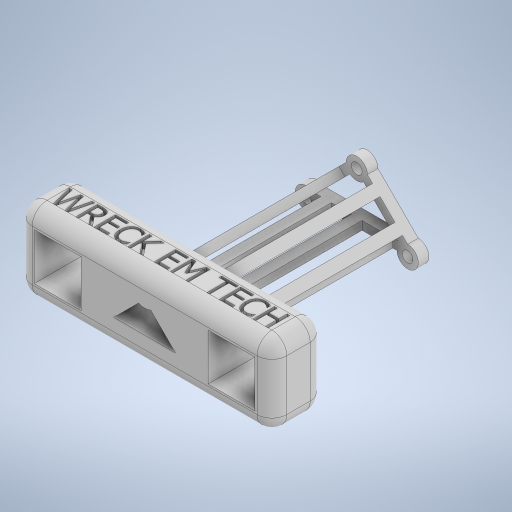
# Autodesk Inventor part: WPNA_FrontHammer
Saved by Autodesk Inventor 2024 (Build 280153000, 153)
## iProperties
Created: 2025-11-09
Part Number: WPNA_FrontHammer
Material: Generic
Document SubType Name: Modeling
Designer: albah
Density: 1 g/cm^3
Appearance: Default
Author: albah
Autodesk Inventor part; units mm, degrees
ref_plane "YZ Plane" through (0, 0, 0) normal (1, 0, 0) x (0, 1, 0)
ref_plane "XZ Plane" through (0, 0, 0) normal (0, 1, 0) x (-1, 0, 0)
sketch "Sketch1" plane through (0, 0, 0) normal (0, 0, 1) x (1, 0, 0)
  line L0 (0, 0) -> (24, 0)
  line L1 (0, 0) -> (-24, 0)
  line L2 (0, 0) -> (0, 24)
  circle A0 centre (0, 24) radius 2.5
  circle A1 centre (24, 0) radius 2.5
  circle A2 centre (-24, 0) radius 2.5
  circle A3 centre (0, 24) radius 5
  circle A4 centre (-24, 0) radius 5
  circle A5 centre (24, 0) radius 5
  line L3 (-24, 5) -> (-5, 24)
  line L4 (5, 24) -> (24, 5)
  line L5 (2.1716, 21.1716) -> (21.1716, 2.1716)
  line L6 (-21.1716, 2.1716) -> (-2.1716, 21.1716)
  line L7 (0, 4) -> (24, 4)
  line L8 (0, 4) -> (-24, 4)
  line L9 (-20.5858, 8.4142) -> (-17.7574, 5.5858)
  line L10 (-17.7574, 5.5858) -> (-14.2218, 9.1213)
  line L11 (-14.2218, 9.1213) -> (-17.0503, 11.9497)
  line L12 (-17.0503, 11.9497) -> (-20.5858, 8.4142)
  line L13 (-11.9497, 17.0503) -> (-9.1213, 14.2218)
  line L14 (-9.1213, 14.2218) -> (-5.5858, 17.7574)
  line L15 (-5.5858, 17.7574) -> (-8.4142, 20.5858)
  line L16 (-8.4142, 20.5858) -> (-11.9497, 17.0503)
  line L17 (7.4497, 21.5503) -> (4.6213, 18.7218)
  line L18 (4.6213, 18.7218) -> (8.1569, 15.1863)
  line L19 (8.1569, 15.1863) -> (10.9853, 18.0147)
  line L20 (10.9853, 18.0147) -> (7.4497, 21.5503)
  line L21 (21.5503, 7.4497) -> (18.7218, 4.6213)
  line L22 (18.7218, 4.6213) -> (15.1863, 8.1569)
  line L23 (15.1863, 8.1569) -> (18.0147, 10.9853)
  line L24 (18.0147, 10.9853) -> (21.5503, 7.4497)
  line L25 (17, 4) -> (17, 0)
  line L26 (17, 0) -> (12, 0)
  line L27 (12, 0) -> (12, 4)
  line L28 (12, 4) -> (17, 4)
  line L29 (1.1005, 0) -> (-3.8995, 0)
  line L30 (-3.8995, 4) -> (1.1005, 4)
  line L31 (-12, 4) -> (-12, 0)
  line L32 (-12, 0) -> (-17, 0)
  line L33 (-17, 0) -> (-17, 4)
  line L34 (-17, 4) -> (-12, 4)
  line L35 (-2.5, 0) -> (2.5, 0)
  line L36 (2.5, 0) -> (2.5, 4)
  line L37 (2.5, 4) -> (-2.5, 4)
  line L38 (-2.5, 4) -> (-2.5, 0)
  line L39 (-2.5, 0) -> (2.5, 4) construction
  line L40 (2.5, 0) -> (-2.5, 4) construction
  point P0 (-7, 19.1716)
  point P1 (-19.1716, 7)
  point P2 (0, 2)
  point P3 (-3.1918, 20.1513)
  point P4 (-19, 0)
  point P5 (19, 0)
  point P6 (3.1918, 20.1513)
  point P7 (19.3431, 4)
  point P8 (-19.3431, 4)
  dimension "d7" = 10
  dimension "d0" = 24
  dimension "d1" = 24
  dimension "d2" = 24
  dimension "d3" = 5
  dimension "d4" = 5
  dimension "d5" = 5
  dimension "d6" = 10
  dimension "d8" = 10
  dimension "d9" = 4
  dimension "d10" = 4
  dimension "d11" = 4
  dimension "d12" = 4
  dimension "d13" = 45
  dimension "d14" = 20.5061
  dimension "d15" = 16.5061
  dimension "d16" = 1
  dimension "d17" = 0.7071
  dimension "d18" = 1.8284
  dimension "d19" = 17.1716
  dimension "d20" = 17.6777
  dimension "d21" = 17.6777
  dimension "d22" = 7.0711
  dimension "d23" = 33.9411
  dimension "d24" = 34.6482
  dimension "d27" = 5
  dimension "d28" = 5
  dimension "d29" = 5
  dimension "d30" = 5
  dimension "d31" = 5
  dimension "d32" = 5
  dimension "d33" = 5
  dimension "d34" = 7
  dimension "d35" = 7
  dimension "d36" = 7
  dimension "d37" = 7
  dimension "d38" = 5
  dimension "d39" = 7
  dimension "d40" = 7
  dimension "d41" = 6.34
  dimension "d42" = 135
  dimension "d43" = 0
  dimension "d44" = 9.1924
  dimension "d45" = 15.5564
  constraints: 82 end point, 19 parallel, 15 perpendicular, 14 point on line, 6 coincident, 6 midpoint, 5 centre point, 2 horizontal, 2 point on circle, 1 vertical, 3 other
  measures "d0" distance of L0.start L0.end
  measures "d1" distance of L0.start L1.end
  measures "d2" distance of L0.start L2.end
  measures "d3" diameter of A0
  measures "d4" diameter of A1
  measures "d5" diameter of A2
  measures "d6" diameter of A3
  measures "d8" diameter of A5
  measures "d9" distance between parallel lines of L4 L5
  measures "d10" distance between parallel lines of L3 L6
  measures "d11" distance between parallel lines of L0 L7
  measures "d12" distance between parallel lines of L1 L8
  measures "d13" angle of L7 L4
  measures "d14" distance from line of L0.start L4
  measures "d15" distance from line of L0.start L6
  measures "d16" distance from line of L4.end L7
  measures "d17" distance from line of L7.end L4
  measures "d18" distance from line of L5.end L7
  measures "d19" distance from line of L5.start L7
  measures "d20" distance from line of L7.start L4
  measures "d21" distance from line of L8.start L4
  measures "d22" distance from line of L6.end L4
  measures "d23" distance from line of L6.start L4
  measures "d24" distance from line of L8.end L4
  measures "d27" distance of L10.end L9.end
  measures "d28" distance of L14.end L13.end
  measures "d29" distance of L18.end L17.end
  measures "d30" distance of L21.end L22.end
  measures "d31" distance of L25.end L26.end
  measures "d32" distance of L29.start L29.end
  measures "d33" distance of L31.end L32.end
  measures "d34" horizontal distance of A3.centre point (-7, 19.172)
  measures "d35" vertical distance of point (-24, 0) point (-19.172, 7)
  measures "d36" distance from line of point (-24, 0) L33
  measures "d37" distance from line of A5.centre L25
  measures "d38" distance of L35.start L35.end
  measures "d39" distance from line of A5.centre L21
  measures "d40" distance from line of A3.centre L17
  measures "d41" angle of L21 L39
  measures "d42" angle of L30 L21
  measures "d43" distance between parallel lines of L7 L37
  measures "d44" distance from line of L29.start L21
  measures "d45" distance from line of L30.start L21
extrude "Extrusion1" add sketch "Sketch1" along normal blind 5 contours L2 L7 L36 L0 | L1 L38 L8 L2 | L1 L31 L8 L38 | L36 L7 L27 L0 | A3 | L27 L7 L25 L0 | L1 L33 L8 L31 | L6 L15 L3 A3 | A3 L4 L17 L5 | L25 L7 L5 A5 L0 | L1 A4 L6 L8 L33 | L6 L13 L3 L15 | L17 L4 L19 L5 | A5 | A4 | L6 L11 L3 L13 | L19 L4 L23 L5 | L5 L7 A5 | L5 L21 L4 A5 L7 | L3 L9 L6 L8 A4 | A4 L8 L6 | L6 L9 L3 L11 | L23 L4 L21 L5
extrude "Extrusion2" add sketch "Sketch1" along normal blind 80 contours L2 L7 L36 L0 | L1 L38 L8 L2 | L27 L7 L25 L0 | L1 L33 L8 L31 | L6 L13 L3 L15 | L17 L4 L19 L5 | L6 L9 L3 L11 | L23 L4 L21 L5
sketch "Sketch2" plane through (0, 0, 80) normal (0, 0, 1) x (1, 0, 0)
  arc A0 (-24, 5) -> (-19, 0) centre (-24, 0) ccw projected
  line L0 (-24, -5) -> (24, -5)
  arc A1 (19, 0) -> (24, 5) centre (24, 0) ccw projected
  line L1 (0, -5) -> (0, 29)
  arc A2 (5, 24) -> (-5, 24) centre (0, 24) ccw projected
  line L2 (-60, -7) -> (60, -7)
  line L3 (60, -7) -> (60, 31)
  line L4 (60, 31) -> (-60, 31)
  line L5 (-60, 31) -> (-60, -7)
  line L6 (-60, -7) -> (60, 31) construction
  line L7 (60, -7) -> (-60, 31) construction
  point P0 (0, 0)
  point P1 (0, 12)
  dimension "d48" = 120
  dimension "d49" = 38
  constraints: 16 end point, 4 midpoint, 3 perpendicular, 3 point on circle, 2 parallel, 2 tangent
  measures "d48" distance of L2.start L2.end
  measures "d49" distance of L3.end L2.end
extrude "Extrusion3" add sketch "Sketch2" along normal blind 25
sketch "Sketch3" plane through (0, 0, 80) normal (0, 0, -1) x (-1, 0, 0)
  line L0 (30, 23) -> (30, 1)
  line L1 (30, 1) -> (52, 1)
  line L2 (52, 1) -> (52, 23)
  line L3 (52, 23) -> (30, 23)
  line L4 (30, 23) -> (52, 1) construction
  line L5 (30, 1) -> (52, 23) construction
  line L6 (60, 31) -> (60, -7) projected
  line L7 (-60, 31) -> (60, 31) projected
  line L8 (60, -7) -> (-60, -7) projected
  line L9 (-52, 23) -> (-30, 23)
  line L10 (-30, 23) -> (-30, 1)
  line L11 (-30, 1) -> (-52, 1)
  line L12 (-52, 1) -> (-52, 23)
  line L13 (-52, 23) -> (-30, 1) construction
  line L14 (-30, 23) -> (-52, 1) construction
  line L15 (-60, -7) -> (-60, 31) projected
  line L16 (-19.3431, 4) -> (19.3431, 4) projected
  line L17 (-3.1918, 20.1513) -> (-4.6213, 18.7218) projected
  line L18 (-3.1918, 20.1513) -> (-19.3431, 4)
  line L19 (-19.3431, 4) -> (19.3431, 4)
  line L20 (19.3431, 4) -> (3.1918, 20.1513)
  arc A0 (-3.1918, 20.1513) -> (3.1918, 20.1513) centre (0, 24) ccw projected
  arc A1 (-3.1918, 20.1513) -> (3.1918, 20.1513) centre (0, 24) ccw
  line L21 (-14.5147, 6) -> (-2.8902, 17.6245)
  arc A2 (-2.8902, 17.6245) -> (2.8902, 17.6245) centre (0, 24) ccw
  line L22 (2.8902, 17.6245) -> (14.5147, 6)
  line L23 (14.5147, 6) -> (-14.5147, 6)
  point P0 (0, 0)
  point P1 (41, 12)
  point P2 (-41, 12)
  point P3 (0, 4)
  point P4 (0, 4)
  dimension "d52" = 8
  dimension "d53" = 8
  dimension "d54" = 8
  dimension "d55" = 8
  dimension "d56" = 8
  dimension "d57" = 8
  dimension "d58" = 30
  dimension "d59" = 30
  dimension "d62" = 2
  constraints: 36 end point, 6 midpoint, 4 parallel, 4 perpendicular, 4 point on circle, 2 centre point, 2 collinear, 1 horizontal, 1 vertical, 3 other
  measures "d52" distance between parallel lines of L6 L2
  measures "d53" distance between parallel lines of L7 L3
  measures "d54" distance between parallel lines of L8 L1
  measures "d55" distance between parallel lines of L8 L11
  measures "d56" distance between parallel lines of L7 L9
  measures "d57" distance between parallel lines of L15 L12
  measures "d58" distance from line of point (0, 4) L0
  measures "d59" distance from line of point (0, 4) L10
  measures "d62" distance between parallel lines of L18 L21
extrude "Extrusion4" cut sketch "Sketch3" against normal blind 25 contours L3 L2 L1 L0 | L9 L10 L11 L12 | L21 A2 L22 L23
fillet "Fillet1" radius 7 12 edges at (60, 12, 80) (0, -7, 80) (-60, 12, 80) (0, 31, 80) (60, -7, 92.5) (0, -7, 105) (-60, -7, 92.5) (-60, 12, 105) (-60, 31, 92.5) (0, 31, 105) (60, 31, 92.5) (60, 12, 105)
fillet "Fillet2" radius 1 25 edges at (6.0355, 20.136, 80) (6.3891, 16.9541, 80) (9.5711, 16.6005, 80) (9.2175, 19.7825, 80) (20.136, 6.0355, 80) (19.7825, 9.2175, 80) (16.6005, 9.5711, 80) (16.9541, 6.3891, 80) (-12, 2, 80) (-14.5, 4, 80) (-17, 2, 80) (17, 2, 80) (14.5, 4, 80) (12, 2, 80) (2.5, 2, 80) (0, 4, 80) (-2.5, 2, 80) (-19.1716, 7, 80) (-15.9896, 7.3536, 80) (-15.636, 10.5355, 80) (-18.818, 10.182, 80) (-10.5355, 15.636, 80) (-7.3536, 15.9896, 80) (-7, 19.1716, 80) (-10.182, 18.818, 80)
ref_plane "Work Plane1" through (-53, 41, 87) normal (0, 1, 0) x (1, 0, 0)
sketch "Sketch7" plane through (-53, 41, 87) normal (0, 1, 0) x (1, 0, 0)
  line L0 (-3.014, -0.6324) -> (108.4129, -0.6324) construction
  line L1 (108.4129, -0.6324) -> (108.4129, -11.6218) construction
  line L2 (108.4129, -11.6218) -> (-3.014, -11.6218) construction
  line L3 (-3.014, -11.6218) -> (-3.014, -0.6324) construction
  line L4 (12.3267, -0.8106) -> (9.8145, -10.8106)
  line L5 (9.8145, -10.8106) -> (8.3234, -10.8106)
  line L6 (8.3234, -10.8106) -> (6.2894, -2.5124)
  line L7 (6.2894, -2.5124) -> (4.3121, -10.8106)
  line L8 (4.3121, -10.8106) -> (2.8372, -10.8106)
  line L9 (2.8372, -10.8106) -> (0.2845, -0.8106)
  line L10 (0.2845, -0.8106) -> (1.6541, -0.8106)
  line L11 (1.6541, -0.8106) -> (3.6638, -9.1008)
  line L12 (3.6638, -9.1008) -> (5.6573, -0.8106)
  line L13 (5.6573, -0.8106) -> (7.0106, -0.8106)
  line L14 (7.0106, -0.8106) -> (9.0203, -9.198)
  line L15 (9.0203, -9.198) -> (11.022, -0.8106)
  line L16 (11.022, -0.8106) -> (12.3267, -0.8106)
  line L17 (21.257, -10.8106) -> (19.5309, -10.8106)
  line L18 (19.5309, -10.8106) -> (16.3704, -6.8317)
  line L19 (16.3704, -6.8317) -> (14.8469, -6.8317)
  line L20 (14.8469, -6.8317) -> (14.8469, -10.8106)
  line L21 (14.8469, -10.8106) -> (13.5179, -10.8106)
  line L22 (13.5179, -10.8106) -> (13.5179, -0.8106)
  line L23 (13.5179, -0.8106) -> (16.0949, -0.8106)
  spline S0 degree 2 poles (16.0949, -0.8106) (16.9539, -0.8106) (18.1127, -0.997) (18.6395, -1.3374) knots 0 0 0 1 2 2 2
  spline S1 degree 2 poles (18.6395, -1.3374) (19.1662, -1.6777) (19.774, -2.7393) (19.774, -3.5254) knots 0 0 0 1 2 2 2
  spline S2 degree 2 poles (19.774, -3.5254) (19.774, -4.6194) (18.6557, -6.1024) (17.6994, -6.4589) knots 0 0 0 1 2 2 2
  line L24 (17.6994, -6.4589) -> (21.257, -10.8106)
  spline S3 degree 2 poles (18.3883, -3.6307) (18.3883, -3.1931) (18.0803, -2.5205) (17.7562, -2.3017) knots 0 0 0 1 2 2 2
  spline S4 degree 2 poles (17.7562, -2.3017) (17.4725, -2.1153) (16.7189, -1.9614) (16.1678, -1.9614) knots 0 0 0 1 2 2 2
  line L25 (16.1678, -1.9614) -> (14.8469, -1.9614)
  line L26 (14.8469, -1.9614) -> (14.8469, -5.7215)
  line L27 (14.8469, -5.7215) -> (16.0139, -5.7215)
  spline S5 degree 2 poles (16.0139, -5.7215) (16.5892, -5.7215) (17.5049, -5.5189) (17.821, -5.2029) knots 0 0 0 1 2 2 2
  spline S6 degree 2 poles (17.821, -5.2029) (18.1127, -4.9273) (18.3883, -4.1494) (18.3883, -3.6307) knots 0 0 0 1 2 2 2
  line L28 (22.0511, -10.8106) -> (22.0511, -0.8106)
  line L29 (22.0511, -0.8106) -> (28.3072, -0.8106)
  line L30 (28.3072, -0.8106) -> (28.3072, -1.9938)
  line L31 (28.3072, -1.9938) -> (23.3801, -1.9938)
  line L32 (23.3801, -1.9938) -> (23.3801, -4.7328)
  line L33 (23.3801, -4.7328) -> (27.975, -4.7328)
  line L34 (27.975, -4.7328) -> (27.975, -5.916)
  line L35 (27.975, -5.916) -> (23.3801, -5.916)
  line L36 (23.3801, -5.916) -> (23.3801, -9.6275)
  line L37 (23.3801, -9.6275) -> (28.3072, -9.6275)
  line L38 (28.3072, -9.6275) -> (28.3072, -10.8106)
  line L39 (28.3072, -10.8106) -> (22.0511, -10.8106)
  spline S7 degree 2 poles (33.6719, -10.9889) (32.6994, -10.9889) (31.0544, -10.3325) (30.4547, -9.6761) knots 0 0 0 1 2 2 2
  spline S8 degree 2 poles (30.4547, -9.6761) (29.855, -9.0278) (29.1986, -7.0829) (29.1986, -5.8187) knots 0 0 0 1 2 2 2
  spline S9 degree 2 poles (29.1986, -5.8187) (29.1986, -4.5627) (29.8388, -2.6988) (30.4466, -2.01) knots 0 0 0 1 2 2 2
  spline S10 degree 2 poles (30.4466, -2.01) (31.0463, -1.3374) (32.6832, -0.6324) (33.6962, -0.6324) knots 0 0 0 1 2 2 2
  spline S11 degree 2 poles (33.6962, -0.6324) (34.1986, -0.6324) (35.0819, -0.7782) (35.4547, -0.8917) knots 0 0 0 1 2 2 2
  spline S12 degree 2 poles (35.4547, -0.8917) (35.7789, -0.997) (36.4515, -1.2969) (36.7837, -1.4751) knots 0 0 0 1 2 2 2
  line L40 (36.7837, -1.4751) -> (36.7837, -3.0797)
  line L41 (36.7837, -3.0797) -> (36.6784, -3.0797)
  spline S13 degree 2 poles (36.6784, -3.0797) (36.5001, -2.9176) (35.949, -2.4638) (35.5519, -2.245) knots 0 0 0 1 2 2 2
  spline S14 degree 2 poles (35.5519, -2.245) (35.1711, -2.0343) (34.2716, -1.7669) (33.6881, -1.7669) knots 0 0 0 1 2 2 2
  spline S15 degree 2 poles (33.6881, -1.7669) (33.0479, -1.7669) (31.9053, -2.2936) (31.4758, -2.7961) knots 0 0 0 1 2 2 2
  spline S16 degree 2 poles (31.4758, -2.7961) (31.0544, -3.3066) (30.5844, -4.8544) (30.5844, -5.8187) knots 0 0 0 1 2 2 2
  spline S17 degree 2 poles (30.5844, -5.8187) (30.5844, -6.8479) (31.0787, -8.3309) (31.5082, -8.8414) knots 0 0 0 1 2 2 2
  spline S18 degree 2 poles (31.5082, -8.8414) (31.9296, -9.3358) (33.056, -9.8382) (33.6881, -9.8382) knots 0 0 0 1 2 2 2
  spline S19 degree 2 poles (33.6881, -9.8382) (34.2635, -9.8382) (35.244, -9.5546) (35.6249, -9.3439) knots 0 0 0 1 2 2 2
  spline S20 degree 2 poles (35.6249, -9.3439) (35.9895, -9.1332) (36.5325, -8.6956) (36.6865, -8.5416) knots 0 0 0 1 2 2 2
  line L42 (36.6865, -8.5416) -> (36.7837, -8.5416)
  line L43 (36.7837, -8.5416) -> (36.7837, -10.1299)
  spline S21 degree 2 poles (36.7837, -10.1299) (36.4515, -10.2839) (35.868, -10.5675) (35.4547, -10.6972) knots 0 0 0 1 2 2 2
  spline S22 degree 2 poles (35.4547, -10.6972) (35.0171, -10.8431) (34.2716, -10.9889) (33.6719, -10.9889) knots 0 0 0 1 2 2 2
  line L44 (45.3169, -10.8106) -> (43.5908, -10.8106)
  line L45 (43.5908, -10.8106) -> (39.9361, -6.1591)
  line L46 (39.9361, -6.1591) -> (39.3526, -6.8155)
  line L47 (39.3526, -6.8155) -> (39.3526, -10.8106)
  line L48 (39.3526, -10.8106) -> (38.0236, -10.8106)
  line L49 (38.0236, -10.8106) -> (38.0236, -0.8106)
  line L50 (38.0236, -0.8106) -> (39.3526, -0.8106)
  line L51 (39.3526, -0.8106) -> (39.3526, -5.4055)
  line L52 (39.3526, -5.4055) -> (43.4531, -0.8106)
  line L53 (43.4531, -0.8106) -> (45.0738, -0.8106)
  line L54 (45.0738, -0.8106) -> (40.9328, -5.2758)
  line L55 (40.9328, -5.2758) -> (45.3169, -10.8106)
  line L56 (50.4061, -10.8106) -> (50.4061, -0.8106)
  line L57 (50.4061, -0.8106) -> (56.6622, -0.8106)
  line L58 (56.6622, -0.8106) -> (56.6622, -1.9938)
  line L59 (56.6622, -1.9938) -> (51.7351, -1.9938)
  line L60 (51.7351, -1.9938) -> (51.7351, -4.7328)
  line L61 (51.7351, -4.7328) -> (56.3299, -4.7328)
  line L62 (56.3299, -4.7328) -> (56.3299, -5.916)
  line L63 (56.3299, -5.916) -> (51.7351, -5.916)
  line L64 (51.7351, -5.916) -> (51.7351, -9.6275)
  line L65 (51.7351, -9.6275) -> (56.6622, -9.6275)
  line L66 (56.6622, -9.6275) -> (56.6622, -10.8106)
  line L67 (56.6622, -10.8106) -> (50.4061, -10.8106)
  line L68 (66.6946, -10.8106) -> (65.3656, -10.8106)
  line L69 (65.3656, -10.8106) -> (65.3656, -2.1964)
  line L70 (65.3656, -2.1964) -> (62.7562, -8.0554)
  line L71 (62.7562, -8.0554) -> (61.9458, -8.0554)
  line L72 (61.9458, -8.0554) -> (59.3607, -2.1964)
  line L73 (59.3607, -2.1964) -> (59.3607, -10.8106)
  line L74 (59.3607, -10.8106) -> (58.1208, -10.8106)
  line L75 (58.1208, -10.8106) -> (58.1208, -0.8106)
  line L76 (58.1208, -0.8106) -> (59.9361, -0.8106)
  line L77 (59.9361, -0.8106) -> (62.432, -6.3779)
  line L78 (62.432, -6.3779) -> (64.8469, -0.8106)
  line L79 (64.8469, -0.8106) -> (66.6946, -0.8106)
  line L80 (66.6946, -0.8106) -> (66.6946, -10.8106)
  line L81 (75.3494, -10.8106) -> (75.3494, -1.9938)
  line L82 (75.3494, -1.9938) -> (71.9944, -1.9938)
  line L83 (71.9944, -1.9938) -> (71.9944, -0.8106)
  line L84 (71.9944, -0.8106) -> (80.0333, -0.8106)
  line L85 (80.0333, -0.8106) -> (80.0333, -1.9938)
  line L86 (80.0333, -1.9938) -> (76.6784, -1.9938)
  line L87 (76.6784, -1.9938) -> (76.6784, -10.8106)
  line L88 (76.6784, -10.8106) -> (75.3494, -10.8106)
  line L89 (81.0463, -10.8106) -> (81.0463, -0.8106)
  line L90 (81.0463, -0.8106) -> (87.3024, -0.8106)
  line L91 (87.3024, -0.8106) -> (87.3024, -1.9938)
  line L92 (87.3024, -1.9938) -> (82.3753, -1.9938)
  line L93 (82.3753, -1.9938) -> (82.3753, -4.7328)
  line L94 (82.3753, -4.7328) -> (86.9701, -4.7328)
  line L95 (86.9701, -4.7328) -> (86.9701, -5.916)
  line L96 (86.9701, -5.916) -> (82.3753, -5.916)
  line L97 (82.3753, -5.916) -> (82.3753, -9.6275)
  line L98 (82.3753, -9.6275) -> (87.3024, -9.6275)
  line L99 (87.3024, -9.6275) -> (87.3024, -10.8106)
  line L100 (87.3024, -10.8106) -> (81.0463, -10.8106)
  spline S23 degree 2 poles (92.667, -10.9889) (91.6946, -10.9889) (90.0495, -10.3325) (89.4498, -9.6761) knots 0 0 0 1 2 2 2
  spline S24 degree 2 poles (89.4498, -9.6761) (88.8502, -9.0278) (88.1938, -7.0829) (88.1938, -5.8187) knots 0 0 0 1 2 2 2
  spline S25 degree 2 poles (88.1938, -5.8187) (88.1938, -4.5627) (88.834, -2.6988) (89.4417, -2.01) knots 0 0 0 1 2 2 2
  spline S26 degree 2 poles (89.4417, -2.01) (90.0414, -1.3374) (91.6784, -0.6324) (92.6913, -0.6324) knots 0 0 0 1 2 2 2
  spline S27 degree 2 poles (92.6913, -0.6324) (93.1938, -0.6324) (94.0771, -0.7782) (94.4498, -0.8917) knots 0 0 0 1 2 2 2
  spline S28 degree 2 poles (94.4498, -0.8917) (94.774, -0.997) (95.4466, -1.2969) (95.7789, -1.4751) knots 0 0 0 1 2 2 2
  line L101 (95.7789, -1.4751) -> (95.7789, -3.0797)
  line L102 (95.7789, -3.0797) -> (95.6735, -3.0797)
  spline S29 degree 2 poles (95.6735, -3.0797) (95.4952, -2.9176) (94.9442, -2.4638) (94.5471, -2.245) knots 0 0 0 1 2 2 2
  spline S30 degree 2 poles (94.5471, -2.245) (94.1662, -2.0343) (93.2667, -1.7669) (92.6832, -1.7669) knots 0 0 0 1 2 2 2
  spline S31 degree 2 poles (92.6832, -1.7669) (92.043, -1.7669) (90.9004, -2.2936) (90.4709, -2.7961) knots 0 0 0 1 2 2 2
  spline S32 degree 2 poles (90.4709, -2.7961) (90.0495, -3.3066) (89.5795, -4.8544) (89.5795, -5.8187) knots 0 0 0 1 2 2 2
  spline S33 degree 2 poles (89.5795, -5.8187) (89.5795, -6.8479) (90.0738, -8.3309) (90.5033, -8.8414) knots 0 0 0 1 2 2 2
  spline S34 degree 2 poles (90.5033, -8.8414) (90.9247, -9.3358) (92.0511, -9.8382) (92.6832, -9.8382) knots 0 0 0 1 2 2 2
  spline S35 degree 2 poles (92.6832, -9.8382) (93.2586, -9.8382) (94.2391, -9.5546) (94.62, -9.3439) knots 0 0 0 1 2 2 2
  spline S36 degree 2 poles (94.62, -9.3439) (94.9847, -9.1332) (95.5276, -8.6956) (95.6816, -8.5416) knots 0 0 0 1 2 2 2
  line L103 (95.6816, -8.5416) -> (95.7789, -8.5416)
  line L104 (95.7789, -8.5416) -> (95.7789, -10.1299)
  spline S37 degree 2 poles (95.7789, -10.1299) (95.4466, -10.2839) (94.8631, -10.5675) (94.4498, -10.6972) knots 0 0 0 1 2 2 2
  spline S38 degree 2 poles (94.4498, -10.6972) (94.0122, -10.8431) (93.2667, -10.9889) (92.667, -10.9889) knots 0 0 0 1 2 2 2
  line L105 (104.2797, -10.8106) -> (102.9507, -10.8106)
  line L106 (102.9507, -10.8106) -> (102.9507, -5.916)
  line L107 (102.9507, -5.916) -> (98.3477, -5.916)
  line L108 (98.3477, -5.916) -> (98.3477, -10.8106)
  line L109 (98.3477, -10.8106) -> (97.0187, -10.8106)
  line L110 (97.0187, -10.8106) -> (97.0187, -0.8106)
  line L111 (97.0187, -0.8106) -> (98.3477, -0.8106)
  line L112 (98.3477, -0.8106) -> (98.3477, -4.7328)
  line L113 (98.3477, -4.7328) -> (102.9507, -4.7328)
  line L114 (102.9507, -4.7328) -> (102.9507, -0.8106)
  line L115 (102.9507, -0.8106) -> (104.2797, -0.8106)
  line L116 (104.2797, -0.8106) -> (104.2797, -10.8106)
  point P0 (53, 87)
  constraints: 2 other
emboss "Emboss1" sketch "Sketch7" operation cut depth 3 direction (0, -1, 0)
body "Solid1"
